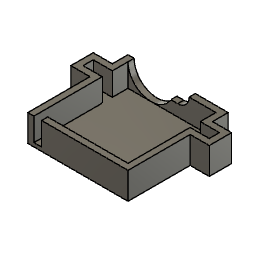
ServoMount (Autodesk Fusion 360 design; units mm, degrees)
Autodesk Fusion 360 part; units mm, degrees
note: some values were not read from the file. Set by a fixed rule: which sketch regions a step uses.
sketch "Sketch1" plane through (0, 0, 0) normal (0, 1, 0) x (1, 0, 0)
  line L0 (0, 0) -> (23, 0)
  line L1 (23, 23) -> (0, 23)
  line L2 (28, 18.9) -> (28, 16.25)
  line L3 (-5, 16.25) -> (-5, 18.9)
  line L4 (-5, 18.9) -> (0, 18.9)
  line L5 (23, 18.9) -> (28, 18.9)
  line L6 (28, 16.25) -> (23, 16.25)
  line L7 (0, 16.25) -> (-5, 16.25)
  line L8 (23, 0) -> (23, 16.25)
  line L9 (23, 18.9) -> (23, 23)
  line L10 (0, 23) -> (0, 18.9)
  line L11 (0, 16.25) -> (0, 0)
  dimension "d1" = 23
  dimension "d2" = 23
  dimension "d3" = 5
  dimension "d4" = 5
  dimension "d5" = 4.1
  dimension "d6" = 6.75
  constraint horizontal L0
  constraint vertical L8
  constraint horizontal L1
  constraint vertical L10
  constraint coincident L0.start L11.end
  constraint horizontal L4
  constraint vertical L2
  constraint horizontal L6
  constraint vertical L3
  constraint coincident L5.start L8
  constraint collinear L4 L5
  constraint coincident L7.start L10
  constraint collinear L6 L7
  constraint collinear L8 L9
  constraint collinear L10 L11
  measures "d1" distance of L0.start L1.end
  measures "d2" distance of L0.start L0.end
  measures "d3" distance of L3 L10
  measures "d4" distance of L2 L8
  measures "d5" distance of L1 L4
  measures "d6" distance of L1 L6
extrude "Extrude1" add sketch "Sketch1" along normal blind 12 makes body 1
sketch "Sketch4" plane through (0, 0, -23) normal (0, 0, -1) x (-1, 0, 0)
  line L0 (-23, 0) -> (0, 0)
  line L1 (0, 0) -> (0, 12)
  line L2 (0, 12) -> (-23, 12)
  line L3 (-23, 12) -> (-23, 0)
  arc A0 (-13, 9) -> (-13, 3) centre (-13, 6) ccw
  arc A1 (-11.1962, 3) -> (-11.1962, 9) centre (-6, 6) ccw
  line L4 (-13, 3) -> (-11.1962, 3)
  line L5 (-13, 9) -> (-11.1962, 9)
  dimension "d28" = 7
  dimension "d30" = 3
  constraint tangent L0 A1
  constraint tangent L1 A1
  constraint tangent L2 A1
  constraint horizontal A1.centre A0.centre
  constraint tangent A0 L4
  constraint horizontal L4
  constraint horizontal L5
  constraint coincident A1.end L5.end
  constraint tangent A0 L5
  measures "d28" distance of A1.centre A0.centre
  measures "d30" radius of A0
extrude "Extrude4" add sketch "Sketch4" along normal blind 4 contours A0 A1 L4 L5 bodies 1
sketch "Sketch2" plane through (0, 0, 0) normal (0, -1, 0) x (1, 0, 0)
  line L0 (0, -16.25) -> (-5, -16.25)
  line L1 (-5, -16.25) -> (-5, -18.9)
  line L2 (-5, -18.9) -> (0, -18.9)
  line L3 (0, -18.9) -> (0, -23)
  line L4 (23, -23) -> (23, -18.9)
  line L5 (23, -18.9) -> (28, -18.9)
  line L6 (28, -18.9) -> (28, -16.25)
  line L7 (28, -16.25) -> (23, -16.25)
  line L8 (23, -16.25) -> (23, 0)
  line L9 (23, 0) -> (0, 0)
  line L10 (0, 0) -> (0, -16.25)
  line L11 (-1.6, 1.6) -> (24.6, 1.6)
  line L12 (29.6, -14.65) -> (29.6, -20.5)
  line L13 (24.6, -24.6) -> (-1.6, -24.6)
  line L14 (-6.6, -20.5) -> (-6.6, -14.65)
  line L15 (29.6, -14.65) -> (24.6, -14.65)
  line L16 (24.6, -14.65) -> (24.6, 1.6)
  line L17 (24.6, -24.6) -> (24.6, -20.5)
  line L18 (24.6, -20.5) -> (29.6, -20.5)
  line L19 (-1.6, -24.6) -> (-1.6, -20.5)
  line L20 (-1.6, -20.5) -> (-6.6, -20.5)
  line L21 (-1.6, 1.6) -> (-1.6, -14.65)
  line L22 (-1.6, -14.65) -> (-6.6, -14.65)
  line L23 (0, -23) -> (6, -23)
  line L24 (6, -23) -> (23, -23)
  line L25 (0, 0) -> (0, 1.6)
  line L26 (2, 1.6) -> (2, 0)
  dimension "d10" = 1.6
  dimension "d11" = 1.6
  dimension "d12" = 1.6
  dimension "d13" = 1.6
  dimension "d14" = 1.6
  dimension "d15" = 1.6
  dimension "d16" = 1.6
  dimension "d17" = 1.6
  dimension "d18" = 1.6
  dimension "d19" = 1.6
  dimension "d20" = 1.6
  dimension "d31" = 1.6
  dimension "d32" = 2
  constraint horizontal L11
  constraint vertical L12
  constraint horizontal L13
  constraint vertical L14
  constraint perpendicular L12 L15
  constraint perpendicular L11 L16
  constraint perpendicular L13 L17
  constraint perpendicular L12 L18
  constraint perpendicular L13 L19
  constraint perpendicular L14 L20
  constraint perpendicular L11 L21
  constraint perpendicular L14 L22
  constraint coincident L9.end L10.start
  constraint coincident L11 L25.end
  constraint perpendicular L11 L25
  constraint coincident L11 L26.start
  constraint coincident L9 L26.end
  constraint perpendicular L9 L26
  measures "d10" distance of L6 L12
  measures "d11" distance of L9 L11
  measures "d12" distance of L1 L14
  measures "d13" distance of L2 L20
  measures "d14" distance of L3 L19
  measures "d15" distance of L4 L17
  measures "d16" distance of L5 L18
  measures "d17" distance of L7 L15
  measures "d18" distance of L8 L16
  measures "d19" distance of L0 L22
  measures "d20" distance of L10 L21
  measures "d31" distance of L13 L24
  measures "d32" distance of L25 L26
extrude "Extrude2" add sketch "Sketch2" along normal blind 1 separate body makes body 2
extrude "Extrude3" add sketch "Sketch2" against normal blind 6 separate body contours L0 L1 L2 L3 L4 L5 L6 L7 L8 L9 L10 L11 L12 L13 L14 L15 L16 L17 L18 L19 L20 L21 L22 L23 L24 L25 L26 makes body 3
combine "Combine1" operation add target body 3 tool bodies 2
combine "Combine2" operation cut target body 3 tool bodies 1
equation "d10 = d20"
equation "d11 = d20"
equation "d12 = d20"
equation "d13 = d20"
equation "d14 = d20"
equation "d15 = d20"
equation "d16 = d20"
equation "d17 = d20"
equation "d18 = d20"
equation "d19 = d20"
equation "d31 = d20"
